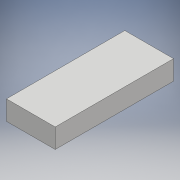
# Autodesk Inventor part: Batery
Saved by Autodesk Inventor 2018 (Build 220112000, 112)
## iProperties
Created: 2017-12-31
Part Number: Batery
Material: Generic
Document SubType Name: Modeling
Designer: suchanek
Density: 1 g/cm^3
Appearance: Default
Author: suchanek
Autodesk Inventor part; units mm, degrees
ref_plane "YZ Plane" through (0, 0, 0) normal (1, 0, 0) x (0, 1, 0)
ref_plane "XZ Plane" through (0, 0, 0) normal (0, 1, 0) x (-1, 0, 0)
ref_plane "XY Plane" through (0, 0, 0) normal (0, 0, 1) x (1, 0, 0)
sketch "Sketch1" plane through (0, 0, 0) normal (0, 1, 0) x (-1, 0, 0)
  line L0 (0, 0) -> (17.5, 0)
  line L1 (17.5, 0) -> (17.5, 7)
  line L2 (17.5, 7) -> (0, 7)
  line L3 (0, 7) -> (0, 0)
  line L4 (17.5, 7) -> (-17.5, 7)
  line L5 (-17.5, 7) -> (-17.5, -7)
  line L6 (-17.5, -7) -> (17.5, -7)
  line L7 (17.5, -7) -> (17.5, 7)
  dimension "d0" = 17.5
  dimension "d1" = 7
  dimension "d2" = 35
  dimension "d3" = 14
  constraints: 16 end point, 4 parallel, 2 horizontal, 2 perpendicular
  measures "d0" distance of L2.end L1.end
  measures "d1" distance of L1.end L0.end
  measures "d2" distance of L6.end L5.end
  measures "d3" distance of L5.end L4.end
extrude "Extrusion1" add sketch "Sketch1" along normal blind 85
body "Solid1"
